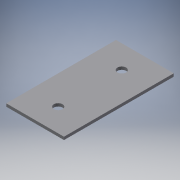
# Autodesk Inventor part: Motor_Plate
Saved by Autodesk Inventor 2017 (Build 210142000, 142)
## iProperties
Created: 2017-11-02
Part Number: Motor_Plate
Material: Generic
Document SubType Name: Modeling
Designer: Aidan_Moga
Density: 1 g/cm^3
Appearance: Default
Mass: 194.596 g
Surface Area: 659.676 cm^2
Volume: 194.596 cm^3
Author: Aidan_Moga
Autodesk Inventor part; units mm, degrees
ref_plane "YZ Plane" through (0, 0, 0) normal (1, 0, 0) x (0, 1, 0)
ref_plane "XZ Plane" through (0, 0, 0) normal (0, 1, 0) x (-1, 0, 0)
ref_plane "XY Plane" through (0, 0, 0) normal (0, 0, 1) x (1, 0, 0)
sketch "Sketch1" plane through (0, 0, 0) normal (0, 1, 0) x (-1, 0, 0)
  line L0 (0, 0) -> (127, 0)
  line L1 (127, 0) -> (127, -241.3)
  line L2 (127, -241.3) -> (0, -241.3)
  line L3 (0, -241.3) -> (0, 0)
  dimension "d0" = 127
  dimension "d1" = 241.3
  constraints: 8 end point, 2 parallel, 1 horizontal, 1 perpendicular
  measures "d0" distance of L1.end L2.end
  measures "d1" distance of L0.end L1.end
extrude "Extrusion1" add sketch "Sketch1" along normal blind 6.35
sketch "Sketch2" plane through (0, 6.35, 0) normal (0, 1, 0) x (1, 0, 0)
  circle A0 centre (-63.5, 50.8) radius 9.525
  circle A1 centre (-63.5, 190.5) radius 9.525
  line L0 (-127, 0) -> (0, 0) projected
  line L1 (0, 241.3) -> (-127, 241.3) projected
  line L2 (-127, 241.3) -> (-127, 0) projected
  dimension "d4" = 19.05
  dimension "d5" = 19.05
  dimension "d6" = 50.8
  dimension "d7" = 50.8
  dimension "d8" = 63.5
  dimension "d9" = 63.5
  constraints: 2 centre point
  measures "d4" diameter of A0
  measures "d5" diameter of A1
  measures "d6" distance from line of L0 A0.centre
  measures "d7" distance from line of L1 A1.centre
  measures "d8" distance from line of L2 A1.centre
  measures "d9" distance from line of L2 A0.centre
extrude "Extrusion2" cut sketch "Sketch2" against normal blind 25.4
body "Solid1"
